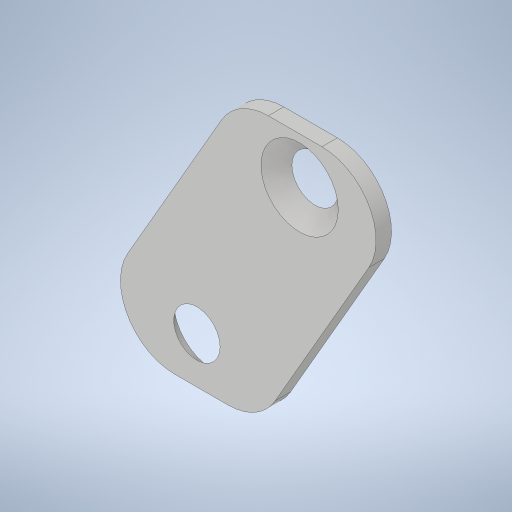
# Autodesk Inventor part: Lamina-02
Saved by Autodesk Inventor 2024.2 (Build 282272000, 272)
## iProperties
Created: 2024-11-25
Part Number: Lamina-02
Material: Genérico
Document SubType Name: Modeling
Designer: jd.castellanosq
Density: 1 g/cm^3
Appearance: Valor por defecto
Author: jd.castellanosq
Autodesk Inventor part; units mm, degrees
ref_plane "YZ Plane" through (0, 0, 0) normal (1, 0, 0) x (0, 1, 0)
ref_plane "XZ Plane" through (0, 0, 0) normal (0, 1, 0) x (-1, 0, 0)
ref_plane "XY Plane" through (0, 0, 0) normal (0, 0, 1) x (1, 0, 0)
sketch "Boceto1" plane through (0, 0, 0) normal (0, 0, 1) x (1, 0, 0)
  line L0 (20.6547, 17.5) -> (0.4474, -17.5)
  line L1 (-22.6466, -17.5) -> (-2.4393, 17.5)
  circle A0 centre (5.6436, 11.5) radius 2.5
  circle A1 centre (-7.6355, -11.5) radius 2.5
  line L2 (-7, 0) -> (7, 0) construction
  line L3 (-2.4393, 17.5) -> (20.6547, 17.5)
  line L4 (-22.6466, -17.5) -> (0.4474, -17.5)
  point P0 (0, 0)
  point P1 (10.5511, 0)
  point P2 (0, 0)
  dimension "d18" = 60
  dimension "d19" = 10
  dimension "d20" = 10
  dimension "d22" = 20
  dimension "d23" = 6
  dimension "d24" = 6
  dimension "d25" = 2.4393
  dimension "d26" = 5
  dimension "d27" = 14
  dimension "d28" = 35
  constraints: 10 end point, 3 horizontal, 2 centre point, 2 coincident, 2 midpoint, 1 equal radius, 1 horizontal alignment, 1 parallel
  measures "d18" angle of L2 L1
  measures "d19" distance from line of L0 A0.centre
  measures "d20" distance from line of L1 A1.centre
  measures "d22" distance between parallel lines of L0 L1
  measures "d23" distance from line of A1.centre L4
  measures "d24" distance from line of L3 A0.centre
  measures "d25" horizontal distance of L1.end point (0, 0)
  measures "d26" diameter of A1
  measures "d27" distance of L2.start L2.end
  measures "d28" distance between parallel lines of L3 L4
extrude "Cuerpo lamina" add sketch "Boceto1" along normal blind 2
fillet "R7" radius 7 4 edges at (20.6547, 17.5, 1) (-2.4393, 17.5, 1) (0.4474, -17.5, 1) (-22.6466, -17.5, 1)
sketch "Boceto3" plane through (0, 0, 0) normal (0, 0, -1) x (-1, 0, 0)
  circle A0 centre (-5.6436, 11.5) radius 2.5 projected
  circle A1 centre (7.6355, -11.5) radius 2.5 projected
  point P0 (0, 0)
hole "BCA M5 Izq" at (-7.6355, -11.5, 0) direction (0, 0, 1) diameter 4.134 depth 14.2 tip angle 118 countersink diameter 10 countersink angle 90 thread size "M5x0.8" class "6H" standard "ANSI Metric M Profile"
sketch "Sketch4" plane through (0, 0, 2) normal (0, 0, 1) x (1, 0, 0)
  circle A0 centre (5.6436, 11.5) radius 2.5 projected
  circle A1 centre (-7.6355, -11.5) radius 2.5 projected
  point P0 (0, 0)
  constraints: 2 coincident
hole "BCA M5 Der" at (5.6436, 11.5, 2) direction (0, 0, -1) diameter 5 depth 14.2 tip angle 118 countersink diameter 10 countersink angle 90
equation "\"d19\" = 0.5 * d22"
equation "\"d20\" = d19"
equation "\"d24\" = d23"
